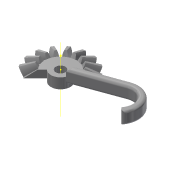
# Autodesk Inventor part: Bevel Gear2
Saved by Autodesk Inventor 2018 (Build 220112000, 112)
## iProperties
Created: 2018-08-06
Part Number: Bevel Gear2
Material: Steel, Mild
Document SubType Name: Modeling
Designer: Bardo91
Categories: <?xml version="1.0" encoding="UTF-16"?> <MemberInstance><Categories><FamilyTemplate><FamilyTemplateParameter ValueType="xs:double" Id="1" ObjectReferenceKey="da_z" ObjectType="kUserParameterObject"/><FamilyTemplateParameter ValueType="xs:double" Id="2" ObjectReferenceKey="da_b" ObjectType="kUserParameterObject"/><FamilyTemplateParameter ValueType="xs:double" Id="3" ObjectReferenceKey="da_beta" ObjectType="kUserParameterObject"/><FamilyTemplateParameter ValueType="xs:double" Id="4" ObjectReferenceKey="da_dae" ObjectType="kUserParameterObject"/><FamilyTemplateParameter ValueType="xs:double" Id="5" ObjectReferenceKey="da_ve" ObjectType="kUserParameterObject"/><FamilyTemplateParameter ValueType="xs:double" Id="6" ObjectReferenceKey="da_omega" ObjectType="kUserParameterObject"/><FamilyTemplateParameter ValueType="xs:string" Id="7" ObjectReferenceKey="EAIAABAAAAAAHwAAAAAAAIAAAAAAAAAA" ObjectType="83914240" SubObjectId="SurfaceGeometry"/></FamilyTemplate><ParamToTemplateMap><ParamToTemplate CategoryParameter="//CategoryParameter[@InternalName='046C89C9-8512-4d59-83FE-43B91F4F132A']" TemplateParameter="1"/><ParamToTemplate CategoryParameter="//CategoryParameter[@InternalName='2552DF32-E462-4b46-AEBF-C6C7768E72AC']" TemplateParameter="2"/><ParamToTemplate CategoryParameter="//CategoryParameter[@InternalName='C9EE641D-15FC-4fae-A226-E94C4372FDD7']" TemplateParameter="3"/><ParamToTemplate><ParamToTemplate CategoryParameter="//CategoryParameter[@InternalName='00B6519A-459B-49c7-AD84-2E56D39A5744']" ConstantValue="-0.350000"/></ParamToTemplate><ParamToTemplate><ParamToTemplate CategoryParameter="//CategoryParameter[@InternalName='04B31F0E-C7A6-4894-AA32-9629BEFACF47']" ConstantValue="1.000000"/></ParamToTemplate><ParamToTemplate><ParamToTemplate CategoryParameter="//CategoryParameter[@InternalName='43CBEC2E-7847-49e7-A936-2F7889FCB2D9']" ConstantValue="0.200000"/></ParamToTemplate><ParamToTemplate><ParamToTemplate CategoryParameter="//CategoryParameter[@InternalName='B1EFC894-105D-4ebd-86BF-FA20ED196853']" ConstantValue="0.300000"/></ParamToTemplate><ParamToTemplate><ParamToTemplate CategoryParameter="//CategoryParameter[@InternalName='51175063-3D10-4879-93E8-6246FE8B403D']" ConstantValue="2060000000.000000"/></ParamToTemplate><ParamToTemplate><ParamToTemplate CategoryParameter="//CategoryParameter[@InternalName='A3A52E27-4454-46a9-B0BD-C932399B70AF']" ConstantValue="0.300000"/></ParamToTemplate><ParamToTemplate CategoryParameter="//CategoryParameter[@InternalName='2A200944-5A8C-41ca-B96E-8520D2E510F1']" TemplateParameter="4"/><ParamToTemplate><ParamToTemplate CategoryParameter="//CategoryParameter[@InternalName='1A637F62-92C8-44bc-B81F-10802510B579']" ConstantValue="2.788931"/></ParamToTemplate><ParamToTemplate CategoryParameter="//CategoryParameter[@InternalName='B52DD4BE-6863-48fb-BF58-89EF6F9EC65C']" TemplateParameter="5"/><ParamToTemplate><ParamToTemplate CategoryParameter="//CategoryParameter[@InternalName='3956BFF2-84D2-457d-93C2-9B0613DEBA67']" ConstantValue="0.575001"/></ParamToTemplate><ParamToTemplate CategoryParameter="//CategoryParameter[@InternalName='739CFA02-461B-4bf8-8049-181FCAD8B28F']" TemplateParameter="6"/><ParamToTemplate><ParamToTemplate CategoryParameter="//CategoryParameter[@InternalName='A27E999F-E2CE-4481-8A2A-EBF499C4C3C5']" ConstantValue="-0.000000"/></ParamToTemplate><ParamToTemplate><ParamToTemplate CategoryParameter="//CategoryParameter[@InternalName='9E1B4470-B2D3-4ff1-B813-535BB4CDF51A']" ConstantValue="3520000.000000"/></ParamToTemplate><ParamToTemplate><ParamToTemplate CategoryParameter="//CategoryParameter[@InternalName='F8452263-BFF6-458c-9FB1-07C4B99E95CD']" ConstantValue="11400000.000000"/></ParamToTemplate><ParamToTemplate><ParamToTemplate CategoryParameter="//CategoryParameter[@InternalName='3E3BB259-FD49-497f-8171-6EBC954A3479']" ConstantValue="2.000000"/></ParamToTemplate><ParamToTemplate CategoryParameter="//CategoryParameter[@InternalName='27C3BAF2-7550-4e4b-AE2C-0DB134B7D9B7']" TemplateParameter="7"/></ParamToTemplateMap><Category DisplayName="Gear" InternalName="DC85795E-93AB-48d5-8EEE-5A27447B64BD" Mnemonic="Gear"><CategoryParameter DisplayName="z" InternalName="046C89C9-8512-4d59-83FE-43B91F4F132A" Mnemonic="z"/><CategoryParameter DisplayName="b" InternalName="2552DF32-E462-4b46-AEBF-C6C7768E72AC" Mnemonic="b"/><CategoryParameter DisplayName="||b|" InternalName="C9EE641D-15FC-4fae-A226-E94C4372FDD7" Mnemonic="beta"/><CategoryParameter DisplayName="x" InternalName="00B6519A-459B-49c7-AD84-2E56D39A5744" Mnemonic="x"/><CategoryParameter DisplayName="a*" InternalName="04B31F0E-C7A6-4894-AA32-9629BEFACF47" Mnemonic="a"/><CategoryParameter DisplayName="c*" InternalName="43CBEC2E-7847-49e7-A936-2F7889FCB2D9" Mnemonic="c"/><CategoryParameter DisplayName="r|.f|*" InternalName="B1EFC894-105D-4ebd-86BF-FA20ED196853" Mnemonic="rf"/><CategoryParameter DisplayName="E" InternalName="51175063-3D10-4879-93E8-6246FE8B403D" Mnemonic="E"/><CategoryParameter DisplayName="||m|" InternalName="A3A52E27-4454-46a9-B0BD-C932399B70AF" Mnemonic="mi"/><Category DisplayName="BevelGear" InternalName="0C98F69A-0C2B-4791-B2FE-7691BB227E77" Mnemonic="BevelGear"><CategoryParameter DisplayName="d|.ae|" InternalName="2A200944-5A8C-41ca-B96E-8520D2E510F1" Mnemonic="dae"/><CategoryParameter DisplayName="d|.ai|" InternalName="1A637F62-92C8-44bc-B81F-10802510B579" Mnemonic="dai"/><CategoryParameter DisplayName="A|.e|" InternalName="B52DD4BE-6863-48fb-BF58-89EF6F9EC65C" Mnemonic="ve"/><CategoryParameter DisplayName="A|.i|" InternalName="3956BFF2-84D2-457d-93C2-9B0613DEBA67" Mnemonic="vi"/><CategoryParameter DisplayName="||S|" InternalName="739CFA02-461B-4bf8-8049-181FCAD8B28F" Mnemonic="omega"/><CategoryParameter DisplayName="x|.t|" InternalName="A27E999F-E2CE-4481-8A2A-EBF499C4C3C5" Mnemonic="xt"/><CategoryParameter DisplayName="||s||.Flim|" InternalName="9E1B4470-B2D3-4ff1-B813-535BB4CDF51A" Mnemonic="sFlim"/><CategoryParameter DisplayName="||s||.Hlim|" InternalName="F8452263-BFF6-458c-9FB1-07C4B99E95CD" Mnemonic="sHlim"/><CategoryParameter DisplayName="type" InternalName="3E3BB259-FD49-497f-8171-6EBC954A3479" Mnemonic="type"/><CategoryParameter DisplayName="PitchDiameter" InternalName="27C3BAF2-7550-4e4b-AE2C-0DB134B7D9B7" Mnemonic="IDS_PITCHDIAM"/></Category></Category></Categories></MemberInstance>
Mass: 60.9118 g
Surface Area: 34.3074 cm^2
Volume: 7.7496 cm^3
Density: 7.86 g/cm^3
Appearance: Steel
CustomPartVersion: 1
Author: Bardo91
Autodesk Inventor part; units mm, degrees
ref_plane "Mesh Plane2" through (0, 0, 0) normal (0.9807853, 0.1950903, 0) x (0, 0, 1)
sketch "Teeth Body Sketch" plane through (0, 0, 0) normal (1, 0, 0) x (0, 1, 0)
  line L0 (0, 0) -> (20.4591, -15.0818) construction
  line L1 (20.4591, -15.0818) -> (23.2139, -9.5721)
  line L2 (23.2139, -9.5721) -> (0, 0) construction
  line L3 (22.4, -11.2) -> (0, 0) construction
  line L4 (12.2898, -9.0597) -> (13.9447, -5.75)
  line L5 (20.4591, -15.0818) -> (12.2898, -9.0597)
  line L6 (23.2139, -9.5721) -> (13.9447, -5.75)
  line L7 (0, -18.0982) -> (0, 3.0164) projected
  line L8 (0, -11.2) -> (23.2139, -11.2) construction
  dimension "d0" = 44.8
  dimension "d1" = 40.9182
  dimension "d2" = 46.4279
  dimension "d3" = 10
  dimension "d4" = 9.5721
  constraints: 16 end point, 4 point on line, 3 perpendicular, 2 collinear, 1 horizontal alignment, 1 vertical alignment
  measures "d0" diameter of L3.start L7
  measures "d1" diameter of L0.end L7
  measures "d2" diameter of L1.end L7
  measures "d3" distance between parallel lines of L1 L4
  measures "d4" vertical distance of L1.end L0.start
revolve "Teeth Body" add sketch "Teeth Body Sketch" angle 360 about axis through (0, 0, 0) along (0, 0, 1)
ref_plane "Tooth Plane" through (0, 22.4, -11.2) normal (0, -0.8944272, 0.4472136) x (1, 0, 0)
sketch "Start Sketch" plane through (0, 22.4, -11.2) normal (0, -0.8944272, 0.4472136) x (1, 0, 0)
  line L0 (0, -60.8499) -> (0, 14.4836) projected
  arc A0 (-1.3526, -5.0792) -> (-4.6853, 3.4634) centre (-16.4663, -6.0541) ccw
  arc A1 (4.6853, 3.4634) -> (1.3526, -5.0792) centre (16.4663, -6.0541) ccw
  line L1 (-1.3526, -5.0792) -> (1.3526, -5.0792)
  arc A2 (4.6853, 3.4634) -> (-4.6853, 3.4634) centre (0, -50.0879) ccw
  dimension "d7" = 15.1451
  dimension "d8" = 16.4663
  dimension "d9" = 44.0338
  dimension "d57" = 53.7559
  dimension "d58" = 45.0087
  constraints: 6 point on circle, 3 centre point, 3 symmetric about line, 2 end point, 1 coincident, 1 perpendicular, 1 other
  measures "d7" radius of A0
  measures "d8" horizontal distance of point (0, -50.088) A0.centre
  measures "d9" vertical distance of point (0, -50.088) A0.centre
  measures "d57" radius of A2
  measures "d58" distance from line of A2.centre L1
sketch "End Sketch" plane through (0, 13.1802, -6.5901) normal (0, -0.8944272, 0.4472136) x (1, 0, 0)
  line L0 (0, -35.815) -> (0, 8.5868) projected
  arc A0 (-0.7972, -2.9436) -> (-2.7615, 2.0914) centre (-9.7053, -3.5182) ccw
  arc A1 (2.7615, 2.0914) -> (0.7972, -2.9436) centre (9.7053, -3.5182) ccw
  line L1 (-0.7972, -2.9436) -> (0.7972, -2.9436)
  arc A2 (2.7615, 2.0914) -> (-2.7615, 2.0914) centre (0, -29.4719) ccw
  dimension "d12" = 8.9266
  dimension "d15" = 9.7053
  dimension "d16" = 25.9537
  dimension "d59" = 31.6839
  dimension "d60" = 26.5283
  constraints: 6 point on circle, 3 centre point, 3 symmetric about line, 2 end point, 1 coincident, 1 other
  measures "d12" radius of A0
  measures "d15" horizontal distance of A0.centre point (0, -29.472)
  measures "d16" vertical distance of A0.centre point (0, -29.472)
  measures "d59" radius of A2
  measures "d60" distance from line of A2.centre L1
loft "Loft" cut profiles "Start Sketch", "End Sketch"
pattern_circular "Circular Pattern" count 16 over 360 about axis through (0, 0, 0) along (0, 0, 1) of "Loft"
ref_plane "End Plane" through (0, 13.1802, -6.5901) normal (0, -0.8944272, 0.4472136) x (1, 0, 0)
sketch3d "3D Sketch Right"
ref_plane "End Plane Right" through (-2.7382, 12.8927, -6.5901) normal (0.1858156, -0.8749129, 0.4472136) x (0.9781824, 0.2077481, 0)
sketch "End Sketch Right" plane through (-2.7382, 12.8927, -6.5901) normal (0.1858156, -0.8749129, 0.4472136) x (0.9781824, 0.2077481, 0)
  arc A0 (-0.7972, -2.9436) -> (-2.7615, 2.0914) centre (-9.7053, -3.5182) ccw
  line L0 (0, -38.2847) -> (0, 11.0565) projected
  arc A1 (2.7615, 2.0914) -> (0.7972, -2.9436) centre (9.7053, -3.5182) ccw
  line L1 (-0.7972, -2.9436) -> (0.7972, -2.9436)
  arc A2 (2.7615, 2.0914) -> (-2.7615, 2.0914) centre (0, -29.4719) ccw
  dimension "d70" = 9.7053
  dimension "d71" = 25.9537
  dimension "d72" = 8.9266
  dimension "d73" = 26.5283
  dimension "d74" = 31.6839
  constraints: 6 point on circle, 3 centre point, 3 symmetric about line, 2 end point, 1 coincident, 1 perpendicular, 1 other
  measures "d70" horizontal distance of A2.centre A0.centre
  measures "d71" vertical distance of point (0, -29.472) A0.centre
  measures "d72" radius of A0
  measures "d73" distance from line of point (0, -29.472) L1
  measures "d74" radius of A2
feature "Loft Right" [suppressed]
pattern_circular "Circular Pattern Right" [suppressed]
sketch3d "3D Sketch Left"
ref_plane "End Plane Left" through (2.8067, 12.8927, -6.6315) normal (-0.1900619, -0.8730501, 0.4490657) x (0.977114, -0.2127164, 0)
sketch "End Sketch Left" plane through (2.8067, 12.8927, -6.6315) normal (-0.1900619, -0.8730501, 0.4490657) x (0.977114, -0.2127164, 0)
  line L0 (0, -39.4288) -> (0, 12.2618) projected
  arc A0 (-0.7972, -2.913) -> (-2.7615, 2.122) centre (-9.7053, -3.4877) ccw
  arc A1 (2.7615, 2.122) -> (0.7972, -2.913) centre (9.7053, -3.4877) ccw
  line L1 (-0.7972, -2.913) -> (0.7972, -2.913)
  ellipse E0 centre (0, -5.1376) end of major axis (13.9447, -5.1376) minor radius 6.2621 projected
  arc A2 (2.7615, 2.122) -> (-2.7615, 2.122) centre (0, -29.4413) ccw
  dimension "d56" = 6.2621
  dimension "d30" = 8.9266
  dimension "d31" = 9.7053
  dimension "d32" = 25.9537
  dimension "d61" = 31.6839
  dimension "d62" = 26.5283
  constraints: 6 point on circle, 3 centre point, 3 symmetric about line, 2 end point, 1 coincident, 2 other
  measures "d30" radius of A0
  measures "d31" horizontal distance of point (0, -29.441) A0.centre
  measures "d32" vertical distance of A0.centre point (0, -29.441)
  measures "d61" radius of A2
  measures "d62" distance from line of point (0, -29.441) L1
feature "Loft Left" [suppressed]
pattern_circular "Circular Pattern Left" [suppressed]
sketch "Body Sketch" plane through (0, 0, 0) normal (1, 0, 0) x (0, 1, 0)
  line L0 (0, -16.2862) -> (0, -7.8553) projected
  line L1 (20.4591, -15.0818) -> (12.2898, -9.0597) projected
  line L2 (12.2898, -9.0597) -> (0, -9.0597)
  line L3 (20.4591, -15.0818) -> (0, -15.0818)
  constraints: 4 end point, 2 perpendicular, 2 point on line
revolve "Fix Body" add sketch "Body Sketch" angle 360 about axis through (0, 0, 0) along (0, 0, 1)
sketch "Sketch6" plane through (0, 0, 0) normal (1, 0, 0) x (0, 1, 0)
  line L0 (22.4, -11.2) -> (0, 0) projected
  line L1 (0, -13.44) -> (0, 2.24) projected
surface revolve "Pitch Diameter" sketch "Sketch6" angle 360 about axis through (0, 0, 0) along (0, 0, 1) shown no curves L0
sketch "Sketch11" plane through (0, 0, -9.0597) normal (0, 0, 1) x (1, 0, 0)
  arc A0 (-5.3033, -5.3033) -> (7.0477, 2.5652) centre (0, 0) ccw
  arc A1 (-17.6777, -17.6777) -> (23.4923, 8.5505) centre (0, 0) ccw
  line L0 (0, 0) -> (23.4923, 8.5505)
  line L1 (0, 0) -> (25, 0) construction
  line L2 (0, 0) -> (-17.6777, -17.6777)
  line L3 (0, 0) -> (25, 0) construction
  arc A2 (7.0477, 2.5652) -> (-5.3033, -5.3033) centre (0, 0) ccw
  dimension "d108" = 15
  dimension "d109" = 50
  dimension "d110" = 20
  dimension "d111" = 225
  constraints: 8 end point, 6 point on circle, 3 centre point, 2 coincident, 2 horizontal, 2 point on line, 1 equal length
  measures "d108" diameter of A0
  measures "d109" diameter of A1
  measures "d110" angle of L1 L0
extrude "Extrusion3" cut sketch "Sketch11" along normal through all both and the other way through all contours A0 L0 A1 L2
sketch "Sketch12" plane through (0, 0, -15.0818) normal (0, 0, -1) x (-1, 0, 0)
  circle A0 centre (0, 0) radius 3.75
  circle A1 centre (0, 0) radius 7.5
  dimension "d116" = 7.5
  dimension "d117" = 15
  constraints: 2 centre point, 2 coincident
  measures "d116" diameter of A0
  measures "d117" diameter of A1
extrude "Extrusion4" add sketch "Sketch12" along normal blind 2
sketch "Sketch13" plane through (0, 0, -9.0597) normal (0, 0, 1) x (1, 0, 0)
  point P0 (0, 0)
sketch "Sketch14" plane through (0, 0, -9.0597) normal (0, 0, 1) x (1, 0, 0)
  arc A0 (-5.3033, -5.3033) -> (7.0477, 2.5652) centre (0, 0) ccw projected
  line L0 (7.0477, 2.5652) -> (39.9369, 14.5359)
  line L1 (11.5487, 4.2034) -> (19.2253, 6.9974) projected
  line L2 (39.9369, 14.5359) -> (45.0672, 0.4405)
  arc A1 (56.5579, -9.2013) -> (39.9369, 14.5359) centre (45.0672, 0.4405) ccw
  line L3 (45.0672, 0.4405) -> (56.5579, -9.2013)
  line L4 (45.0672, 0.4405) -> (60.0672, 0.4405) construction
  arc A2 (52.7277, -5.9874) -> (41.647, 9.8374) centre (45.0672, 0.4405) ccw
  line L5 (41.647, 9.8374) -> (6.9631, -2.7865)
  dimension "d118" = 35
  dimension "d119" = 15
  dimension "d120" = 40
  dimension "d121" = 20
  dimension "d127" = 5
  constraints: 10 end point, 5 point on circle, 2 centre point, 2 coincident, 2 point on line, 1 collinear, 1 equal length, 1 horizontal, 1 parallel
  measures "d118" distance of L0.start L0.end
  measures "d119" distance of L0.end L2.end
  measures "d120" angle of L3 L4
  measures "d121" diameter of A2
  measures "d127" distance between parallel lines of L5 L0
extrude "Extrusion5" add sketch "Sketch14" along normal mid plane 10 contours A0 L0 L2 L5 | L2 A1 L3 A2
sketch "Sketch8" plane through (0, 0, -9.0597) normal (0, 0, 1) x (1, 0, 0)
  circle A0 centre (0, 0) radius 3.75
  dimension "d94" = 7.5
  constraints: 1 centre point, 1 coincident
  measures "d94" diameter of A0
extrude "Extrusion1" cut sketch "Sketch8" against normal blind 10
fillet "Fillet1" radius 2 9 edges at (7.4991, -0.1185, -4.0597) (28.9296, 10.5295, -14.0597) (57.3545, 9.0441, -14.0597) (53.2588, 6.1762, -14.0597) (53.2588, 6.1762, -4.0597) (23.4923, 8.5505, -4.0597) (57.3545, 9.0441, -4.0597) (56.5579, -9.2013, -9.0597) (52.7277, -5.9874, -9.0597)
equation "\"d0\" = da_de"
equation "\"d1\" = da_dfe"
equation "\"d2\" = da_dae"
equation "\"d3\" = da_b"
equation "\"d4\" = da_ve"
equation "\"d7\" = fd_rr"
equation "\"d8\" = fd_x"
equation "\"d9\" = fd_y"
equation "\"d57\" = 0.5 * fd_dva + 0.3 * da_he"
equation "\"d58\" = 0.5 * fd_dva - 1.12 * da_he"
equation "\"da_teethtype\" = 0"
equation "\"da_b\" = 10"
equation "\"da_de\" = 44.8"
equation "\"da_dae\" = 46.42786"
equation "\"da_dfe\" = 40.91819"
equation "\"da_le\" = 25.04396"
equation "\"da_omega\" = 90deg"
equation "\"da_beta\" = 0"
equation "\"da_delta\" = 63.434949deg"
equation "\"da_alpha\" = 20deg"
equation "\"da_he\" = 6.16"
equation "\"da_ve\" = 9.57214"
equation "\"da_zv\" = 35.777088"
equation "\"fd_loft\" = da_b + 0.05 * da_he"
equation "\"fd_x\" = fd_x1 + fd_x2"
equation "\"fd_y\" = fd_y1 - fd_y2"
equation "\"fd_dd\" = fd_dva - 0.8 * da_he"
equation "\"da_dvw\" = 98.21585"
equation "\"d11\" = fd_loft"
equation "\"da_dm\" = 35.85573"
equation "\"da_x\" = -0.35"
equation "\"da_m\" = 2.8"
equation "\"d50\" = da_omega"
equation "\"fd_rr\" = 15.145143"
equation "\"fd_dva\" = 103.815845"
equation "\"fd_x1\" = 2.179328"
equation "\"fd_x2\" = 14.286954"
equation "\"fd_y1\" = 49.059541"
equation "\"fd_y2\" = 5.025763"
body "Solid1"
body "Srf1"
